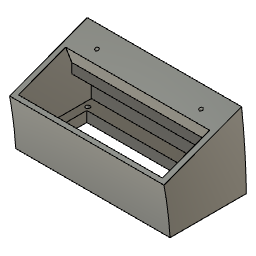
lcd_16_2_ver_3 (Autodesk Fusion 360 design; units mm, degrees)
Autodesk Fusion 360 part; units mm, degrees
note: some values were not read from the file. Chosen so that the rebuilt part matches the saved one: which face or edge a step refers to; which pieces of a blend or face edit are solid. Set by a fixed rule: which sketch regions a step uses.
sketch "Sketch1" plane through (0, 0, 0) normal (0, 0, 1) x (1, 0, 0)
  line L0 (0, 0) -> (82, 0)
  line L1 (82, 0) -> (82, 36)
  line L2 (82, 36) -> (0, 36)
  line L3 (0, 36) -> (0, 0)
  dimension "d1" = 82
  dimension "d2" = 36
  constraint horizontal L0
  constraint vertical L1
  constraint horizontal L2
  constraint vertical L3
  constraint coincident L0.start L3.end
  measures "d1" distance of L0.start L0.end
  measures "d2" distance of L0.start L2.end
extrude "Extrude1" add sketch "Sketch1" along normal blind 25 makes body 1
sketch "Sketch2" plane through (0, 0, 25) normal (0, 0, 1) x (-1, 0, 0)
  line L0 (0, -36) -> (0, 0)
  line L1 (0, 0) -> (-82, 0)
  line L2 (-82, 0) -> (-82, -36)
  line L3 (-82, -36) -> (0, -36)
  line L4 (-3.5, -31.5) -> (-76.5, -31.5)
  line L5 (-76.5, -31.5) -> (-76.5, -4.5)
  line L6 (-76.5, -4.5) -> (-3.5, -4.5)
  line L7 (-3.5, -4.5) -> (-3.5, -31.5)
  dimension "d5" = 73
  dimension "d6" = 27
  dimension "d7" = 3.5
  dimension "d8" = 4.5
  constraint horizontal L4
  constraint vertical L5
  constraint horizontal L6
  constraint vertical L7
  measures "d5" distance of L4.start L4.end
  measures "d6" distance of L4.start L6.end
  measures "d7" distance of L0 L7
  measures "d8" distance of L3 L4
extrude "Extrude2" cut sketch "Sketch2" against normal blind 20 contours L4 L5 L6 L7 bodies 1
sketch "Sketch3" plane through (82, 0, 0) normal (1, 0, 0) x (0, 1, 0)
  line L0 (0, 0) -> (36, 0)
  line L1 (36, 0) -> (36, 25)
  line L2 (36, 25) -> (0, 25)
  line L3 (0, 25) -> (0, 0)
extrude "Extrude3" add 1 faces at (27.3333, 0, 16.6667) along direction (0, -1, 0) blind 2 on bodies 1 bodies 1
extrude "Extrude4" add sketch "Sketch3" 1 faces at (82, 10.6667, 16.6667) along normal blind 2 on bodies 1 bodies 1
extrude "Extrude5" add 1 faces at (56, 36, 8.3333) along direction (0, 1, 0) blind 2 on bodies 1 bodies 1
extrude "Extrude6" add 1 faces at (0, 11.3333, 8.3333) along direction (-1, 0, 0) blind 2 on bodies 1 bodies 1
extrude "Extrude7" cut 1 faces at (27.8333, 13.5, 5) along direction (0, 0, -1) blind 11 on bodies 1 bodies 1
extrude "Extrude8" add 1 faces at (81.5, 22.5, 25) along direction (0, 0, 1) blind 10 on bodies 1 bodies 1
sketch "Sketch4" plane through (0, 0, 35) normal (0, 0, 1) x (-1, 0, 0)
  line L0 (-76.5, -31.5) -> (-76.5, -4.5)
  line L1 (-76.5, -4.5) -> (-3.5, -4.5)
  line L2 (-3.5, -4.5) -> (-3.5, -31.5)
  line L3 (-3.5, -31.5) -> (-76.5, -31.5)
  line L4 (2, 2) -> (-84, 2)
  line L5 (-84, 2) -> (-84, -38)
  line L6 (-84, -38) -> (2, -38)
  line L7 (2, -38) -> (2, 2)
  line L8 (-0.8406, -0.2622) -> (-80.8406, -0.2622)
  line L9 (-80.8406, -0.2622) -> (-80.8406, -36.2622)
  line L10 (-80.8406, -36.2622) -> (-0.8406, -36.2622)
  line L11 (-0.8406, -36.2622) -> (-0.8406, -0.2622)
  dimension "d23" = 80
  dimension "d24" = 36
  constraint horizontal L8
  constraint vertical L9
  constraint horizontal L10
  constraint vertical L11
  measures "d23" distance of L8.start L8.end
  measures "d24" distance of L8.start L10.end
extrude "Extrude9" cut sketch "Sketch4" against normal blind 28 contours L8 L9 L10 L11 bodies 1
sketch "Sketch5" plane through (84, 0, 0) normal (1, 0, 0) x (0, 1, 0)
  line L0 (-2, 0) -> (38, 0)
  line L1 (38, 0) -> (38, 35)
  line L2 (38, 35) -> (-2, 35)
  line L3 (-2, 35) -> (-2, 0)
  line L4 (-2, 35) -> (-2, 20)
  line L5 (38, 35) -> (-2, 20)
  line L6 (-2, 35) -> (38, 35)
  dimension "d27" = 15
  constraint coincident L2.end L3.start
  constraint coincident L3 L4.end
  constraint coincident L1.end L2.start
  measures "d27" distance of L2.end L4.end
extrude "Extrude10" cut sketch "Sketch5" against normal blind 90 contours L2 L3 L4 L5 L6 bodies 1
sketch "Sketch6" plane through (0.8406, 0, 0) normal (1, 0, 0) x (0, 1, 0)
  line L0 (36.2622, 34.3483) -> (0.2622, 20.8483)
  line L1 (0.2622, 20.8483) -> (0.2622, 7)
  line L2 (0.2622, 7) -> (36.2622, 7)
  line L3 (36.2622, 7) -> (36.2622, 34.3483)
sketch "Sketch7" plane through (0.8406, 0, 0) normal (1, 0, 0) x (0, 1, 0)
  line L0 (36.2622, 34.3483) -> (0.2622, 20.8483)
  line L1 (35.8448, 34.1918) -> (26.4815, 30.6806)
  line L2 (26.4815, 25) -> (26.4815, 30.6806)
  line L3 (36.2622, 7) -> (36.2622, 34.3483)
  line L4 (26.4815, 25) -> (36.2622, 28.6677)
  line L5 (36.2622, 34.3483) -> (35.8448, 34.1918)
  dimension "d30" = 10
  constraint coincident L0 L1.start
  constraint coincident L0 L1.end
  constraint vertical L2
  constraint coincident L3 L4.end
  constraint parallel L0 L4
  constraint coincident L0.start L3.end
  measures "d30" distance of L1.start L1.end
extrude "Extrude11" add sketch "Sketch7" along normal blind 80 bodies 1
sketch "Sketch8" plane through (0, -6.8219, 18.1918) normal (0, -0.351123, 0.936329) x (1, 0, 0)
  line L0 (-2, 47.8698) -> (-2, 5.1498)
  line L1 (-2, 5.1498) -> (84, 5.1498)
  line L2 (84, 5.1498) -> (84, 47.8698)
  line L3 (84, 47.8698) -> (-2, 47.8698)
  line L4 (80.8406, 7.5658) -> (0.8406, 7.5658)
  line L5 (0.8406, 7.5658) -> (0.8406, 35.5681)
  line L6 (0.8406, 35.5681) -> (80.8406, 35.5681)
  line L7 (80.8406, 35.5681) -> (80.8406, 7.5658)
sketch "Sketch9" plane through (0, -6.8219, 18.1918) normal (0, -0.351123, 0.936329) x (1, 0, 0)
  circle A0 centre (11, 41.842) radius 1
  line L0 (-2, 47.8698) -> (-2, 5.1498)
  point P0 (71, 41.842)
  dimension "d33" = 2
  dimension "d34" = 13
  measures "d33" diameter of A0
  measures "d34" distance of A0.centre L0
sketch "Sketch10" plane through (0, -6.8219, 18.1918) normal (0, -0.351123, 0.936329) x (1, 0, 0)
  circle A0 centre (71, 41.842) radius 1
  point P0 (71, 41.842)
  dimension "d35" = 2
  constraint coincident P0 A0.centre
  measures "d35" diameter of A0
extrude "Extrude12" cut sketch "Sketch9" against normal blind 6 bodies 1
extrude "Extrude13" cut sketch "Sketch10" against normal blind 6 bodies 1
sketch "Sketch11" plane through (0, 0, 0) normal (0, 0, 1) x (1, 0, 0)
sketch "Sketch12" plane through (0, 0, 0) normal (0, 0, 1) x (1, 0, 0)
  line L0 (-2, -2) -> (84, -2)
sketch "Sketch13" plane through (0, 0, 0) normal (0, 0, -1) x (1, 0, 0)
  line L0 (76.5, -4.5) -> (76.5, -31.5)
  line L1 (76.5, -31.5) -> (3.5, -31.5)
  line L2 (3.5, -31.5) -> (3.5, -4.5)
  line L3 (3.5, -4.5) -> (76.5, -4.5)
  line L4 (-2, -38) -> (84, -38)
  line L5 (84, -38) -> (84, 2)
  line L6 (84, 2) -> (-2, 2)
  line L7 (-2, 2) -> (-2, -38)
  circle A0 centre (2, -1.6) radius 1.25
  line L8 (-2, 2) -> (84, 2)
  circle A1 centre (2, -32.6) radius 1.25
  circle A2 centre (2, -32.6) radius 1.25
  circle A3 centre (77, -32.6) radius 1.25
  circle A4 centre (77, -1.6) radius 1.25
  point P0 (2, -1.6)
  point P1 (2, -32.6)
  point P2 (77, -32.6)
  point P3 (77, -1.6)
  dimension "d42" = 2.5
  dimension "d43" = 4
  dimension "d44" = 3.6
  dimension "d45" = 2.5
  dimension "d46" = 2.5
  dimension "d48" = 2.5
  dimension "d49" = 2.5
  constraint coincident P2 A3.centre
  constraint coincident P3 A4.centre
  measures "d42" diameter of A0
  measures "d43" distance of L7 P0
  measures "d44" distance of P0 L8
  measures "d45" diameter of A1
  measures "d46" diameter of A2
  measures "d48" diameter of A3
  measures "d49" diameter of A4
sketch "Sketch14" plane through (0, 0, 0) normal (0, 0, -1) x (1, 0, 0)
extrude "Extrude14" cut sketch "Sketch13" against normal blind 9 contours L0 L1 A3 | L0 L1 A3 | A0 | A1 A2 | A4 bodies 1
extrude "Extrude15" add 1 faces at (84, 24.6667, 18.3333) along direction (1, 0, 0) blind 1 on bodies 1 bodies 1
extrude "Extrude16" cut 1 faces at (80.8406, 21.002, 13) along direction (1, 0, 0) blind 1 on bodies 1 bodies 1
extrude "Extrude17" add 1 faces at (56, -2, 6.6667) along direction (0, -1, 0) blind 1 on bodies 1 bodies 1
extrude "Extrude18" cut 1 faces at (27.8406, 0.2622, 16.2322) along direction (0, -1, 0) blind 1 on bodies 1 bodies 1
extrude "Extrude19" add 1 faces at (27.8021, 31.5, 4.6667) along direction (0, -1, 0) blind 1 on bodies 1 bodies 1
extrude "Extrude20" cut 1 faces at (82.6749, 22.2947, 0) along direction (0, 0, 1) blind 1 on bodies 1 bodies 1
extrude "Extrude21" cut 1 faces at (0.8406, 20.2272, 14.3333) along direction (-1, 0, 0) blind 1 on bodies 1 bodies 1
extrude "Extrude22" add 1 faces at (-2, 24.6667, 18.6667) along direction (-1, 0, 0) blind 1 on bodies 1 bodies 1
extrude "Extrude23" cut 1 faces at (-0.1594, 20.2272, 14.3333) along direction (-1, 0, 0) blind 1 on bodies 1 bodies 1
extrude "Extrude24" add 1 faces at (-3, 24.6667, 18.6667) along direction (-1, 0, 0) blind 1 on bodies 1 bodies 1
extrude "Extrude25" cut 1 faces at (-0.523, 1.6, 9) along direction (0, 0, -1) blind 2 on bodies 1 bodies 1
extrude "Extrude26" cut 1 faces at (54.1739, 36.2622, 21.4452) along direction (0, 1, 0) blind 1.5 on bodies 1 bodies 1
sketch "Sketch15" plane through (-4, 0, 0) normal (-1, 0, 0) x (0, -1, 0)
  line L0 (-38, 1) -> (3, 1)
  line L1 (3, 1) -> (3, 20)
  line L2 (3, 20) -> (2, 20)
  line L3 (2, 20) -> (-38, 35)
  line L4 (-38, 35) -> (-38, 1)
  line L5 (0, 20.75) -> (2, 20)
  line L6 (3, 19.625) -> (3, 20)
  line L7 (2, 20) -> (3, 19.625)
  constraint coincident L3 L5.start
  constraint coincident L2.end L3.start
  constraint parallel L3 L5
  constraint coincident L1 L6.start
  constraint coincident L1.end L2.start
  constraint perpendicular L2 L6
  constraint parallel L5 L7
extrude "Extrude27" cut sketch "Sketch15" against normal blind 9000 contours L1 L2 L6 L7 bodies 1
extrude "Extrude28" cut 1 faces at (-0.523, 32.6, 9) along direction (0, 0, -1) blind 2 on bodies 1 bodies 1
extrude "Extrude29" add 1 faces at (1.6199, 32.3401, 32.8775) along direction (0, -0.351123, 0.936329) blind 10 on bodies 1 bodies 1
extrude "Extrude45" add 1 faces at (55.3333, 38, 23.6667) along direction (0, 1, 0) blind 3 on bodies 1 bodies 1
extrude "Extrude46" add 1 faces at (25.6667, 40, 35) along direction (0, 0, 1) blind 3 on bodies 1 bodies 1
extrude "Extrude47" cut 1 faces at (25.6667, 36.8296, 38.1211) along direction (0, 0.936329, 0.351123) blind 1 on bodies 1 bodies 1
extrude "Extrude48" cut 1 faces at (25.6667, 36.8296, 38.1211) along direction (0, 0.936329, 0.351123) blind 3 on bodies 1 bodies 1
extrude "Extrude49" add 1 faces at (25.6667, 36.8296, 38.1211) along direction (0, 0.936329, 0.351123) blind 3 on bodies 1 bodies 1
extrude "Extrude50" add 1 faces at (25.6667, 40.386, 38) along direction (0, 0, 1) blind 3 on bodies 1 bodies 1
extrude "Extrude51" cut 1 faces at (55.3333, 38.2248, 42.9444) along direction (0, 0.936329, 0.351123) blind 1 on bodies 1 bodies 1 makes body 2 at (25.6667, 40.693, 39.2107)
extrude "Extrude52" add 1 faces at (55.3333, 38.2248, 42.9444) along direction (0, 0.936329, 0.351123) blind 1 on bodies 1 bodies 1 2
sketch "Sketch17" plane through (-4, 0, 0) normal (-1, 0, 0) x (0, -1, 0)
  line L0 (-41, 38.3454) -> (-41, 1)
  line L1 (-41, 1) -> (3, 1)
  line L2 (3, 1) -> (3, 19.625)
  line L3 (3, 19.625) -> (6.5112, 28.9883)
  line L4 (6.5112, 28.9883) -> (-38.2341, 45.7678)
  line L5 (-38.2341, 45.7678) -> (-40.079, 40.848)
  line L6 (-40.079, 40.848) -> (-40.079, 41)
  line L7 (-40.079, 41) -> (-41, 41)
  line L8 (-41, 41) -> (-41, 38.392)
  line L9 (-41, 38.392) -> (-41.0153, 38.3511)
  line L10 (-41.0153, 38.3511) -> (-41, 38.3454)
  line L11 (-40.079, 41) -> (-38.2341, 45.7678)
  line L12 (-41.104, 38.3511) -> (-41.104, 45.7678)
  line L13 (-40.079, 41) -> (-41, 39.3)
  line L14 (-41, 41) -> (-40.079, 41)
  line L15 (-41, 39.3) -> (-41, 41)
  constraint coincident L6.end L7.start
  constraint coincident L4.end L5.start
  constraint parallel L8 L12
  constraint coincident L8 L13.end
  constraint coincident L7.end L8.start
sketch "Sketch18" plane through (85, 0, 0) normal (1, 0, 0) x (0, 1, 0)
  line L0 (38.2341, 45.7678) -> (-6.5112, 28.9883)
  line L1 (-6.5112, 28.9883) -> (-3, 19.625)
  line L2 (-3, 19.625) -> (-3, 1)
  line L3 (-3, 1) -> (41, 1)
  line L4 (41, 1) -> (41, 38.3454)
  line L5 (41, 38.3454) -> (41.0153, 38.3511)
  line L6 (41.0153, 38.3511) -> (41, 38.392)
  line L7 (41, 38.392) -> (41, 41)
  line L8 (41, 41) -> (40.079, 41)
  line L9 (40.079, 41) -> (40.079, 40.848)
  line L10 (40.079, 40.848) -> (38.2341, 45.7678)
  line L11 (38.2341, 45.7678) -> (41, 34.9623)
  line L12 (41, 45.7022) -> (38.2341, 45.7678)
  constraint coincident L0.start L10.end
  constraint coincident L4 L11.end
extrude "Extrude53" cut sketch "Sketch17" against normal blind 100 contours L7 L8 L13 L14 L15 bodies 1
extrude "Extrude54" cut sketch "Sketch18" against normal blind 100 contours L4 L5 L6 L7 L8 L9 L10 L11 bodies 1
fillet "Fillet7" radius 230 1 edges at (40.5, -3, 19.625) on bodies 1
fillet "Fillet8" radius 510 1 edges at (40.5, 41, 34.9623) on bodies 1
extrude "Extrude38" [suppressed]
extrude "Extrude39" [suppressed]
extrude "Extrude40" [suppressed]
extrude "Extrude41" [suppressed]
extrude "Extrude42" [suppressed]
extrude "Extrude43" [suppressed]
extrude "Extrude44" [suppressed]
fillet "Fillet6" [suppressed]
fillet "Fillet1" [suppressed]
fillet "Fillet2" [suppressed]
extrude "Extrude31" [suppressed]
extrude "Extrude32" [suppressed]
extrude "Extrude33" [suppressed]
extrude "Extrude34" [suppressed]
extrude "Extrude35" [suppressed]
extrude "Extrude36" [suppressed]
sketch "Sketch16" plane through (85, 0, 0) normal (1, 0, 0) x (0, 1, 0)
  line L0 (35, 44.555) -> (-6.5112, 28.9883)
  arc A0 (-3, 1) -> (-6.5112, 28.9883) centre (-123.4966, 0.0976) ccw
  line L1 (-3, 1) -> (41, 1)
  line L2 (41, 1) -> (41, 45.1013)
  line L3 (41, 45.1013) -> (40.6035, 45.1013)
  line L4 (40.6035, 45.1013) -> (41.0861, 45.2823)
  line L5 (41.0861, 45.2823) -> (40.5749, 46.6456)
  line L6 (40.5749, 46.6456) -> (36.4568, 45.1013)
  line L7 (36.4568, 45.1013) -> (35, 45.1013)
  line L8 (35, 45.1013) -> (35, 44.555)
  line L9 (35, 44.555) -> (36.4568, 45.1013)
  constraint coincident L0.start L8.end
  constraint coincident L6.end L7.start
extrude "Extrude37" [suppressed]
fillet "Fillet3" [suppressed]
fillet "Fillet4" [suppressed]
extrude "Extrude30" [suppressed]
fillet "Fillet5" [suppressed]
